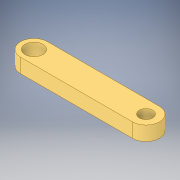
# Autodesk Inventor part: PINZA_ESLABON
Saved by Autodesk Inventor 2019 (Build 230136000, 136)
## iProperties
Created: 2020-02-12
Part Number: PINZA_ESLABON
Material: Genérico
Document SubType Name: Modeling
Designer: omar-
Density: 1 g/cm^3
Appearance: Valor por defecto
Author: omar-
Autodesk Inventor part; units mm, degrees
ref_plane "YZ Plane" through (0, 0, 0) normal (1, 0, 0) x (0, 1, 0)
ref_plane "XZ Plane" through (0, 0, 0) normal (0, 1, 0) x (-1, 0, 0)
ref_plane "XY Plane" through (0, 0, 0) normal (0, 0, 1) x (1, 0, 0)
sketch "Boceto1" plane through (0, 0, 0) normal (0, 1, 0) x (-1, 0, 0)
  line L0 (0, 0) -> (25, 0) construction
  line L1 (0, -3) -> (25, -3)
  line L2 (25, 3) -> (0, 3)
  arc A0 (0, 3) -> (0, -3) centre (0, 0) ccw
  arc A1 (25, -3) -> (25, 3) centre (25, 0) ccw
  circle A2 centre (25, 0) radius 2
  circle A3 centre (0, 0) radius 1.5
  point P0 (12.5, 0)
  dimension "d0" = 25
  dimension "d1" = 6
  dimension "d2" = 4
  dimension "d3" = 3
  constraints: 8 end point, 4 centre point, 4 point on circle, 4 tangent, 2 coincident, 1 horizontal, 1 midpoint, 1 parallel
  measures "d0" distance of L0.start L0.end
  measures "d1" diameter of A1
  measures "d2" diameter of A2
  measures "d3" diameter of A3
extrude "Extrusión1" add sketch "Boceto1" along normal blind 3.18
